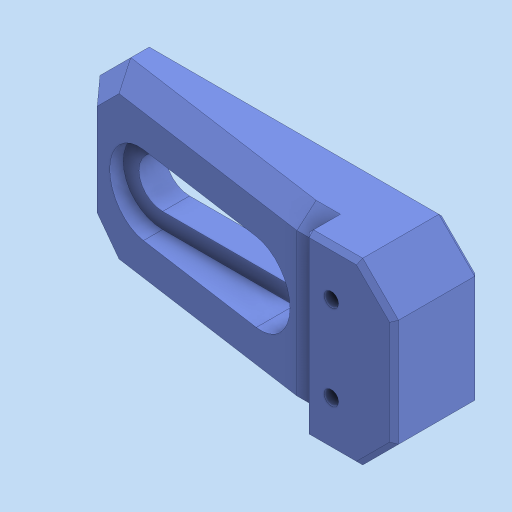
# Autodesk Inventor part: y-Max Endstop Slider for 4040
Saved by Autodesk Inventor 2023.2 (Build 272271000, 271)
## iProperties
Created: 2023-11-28
Part Number: y-Max Endstop Slider for 4040
Material: Generisch
Document SubType Name: Modeling
Designer: Nils Bade
Density: 1 g/cm^3
Appearance: ABS-Blau
Author: Nils Bade
Autodesk Inventor part; units mm, degrees
ref_plane "YZ Plane" through (0, 0, 0) normal (1, 0, 0) x (0, 1, 0)
ref_plane "XZ Plane" through (0, 0, 0) normal (0, 1, 0) x (-1, 0, 0)
ref_plane "XY Plane" through (0, 0, 0) normal (0, 0, 1) x (1, 0, 0)
sketch "S-Base" plane through (0, 0, 0) normal (0, 0, 1) x (1, 0, 0)
  line L0 (-7.35, 0) -> (7.35, 0) construction
  line L1 (-7.35, -2.65) -> (7.35, -2.65)
  line L2 (7.35, 2.65) -> (-7.35, 2.65)
  arc A0 (-7.35, 2.65) -> (-7.35, -2.65) centre (-7.35, 0) ccw
  arc A1 (7.35, -2.65) -> (7.35, 2.65) centre (7.35, 0) ccw
  line L3 (32, 10.3134) -> (32, -10.7721) construction
  line L4 (-24.82, 0) -> (41.47, 0) construction
  circle A2 centre (18, 4.75) radius 0.8
  line L5 (25, 0) -> (25, 10)
  line L6 (25, 10) -> (-15.35, 10)
  line L7 (-15.35, 10) -> (-15.35, 0)
  line L8 (0, 14.5306) -> (0, -14.9892) construction
  line L9 (-7.35, 0) -> (7.35, 0) construction
  line L10 (-7.35, -4.4) -> (7.35, -4.4)
  line L11 (7.35, 4.4) -> (-7.35, 4.4)
  arc A3 (-7.35, 4.4) -> (-7.35, -4.4) centre (-7.35, 0) ccw
  arc A4 (7.35, -4.4) -> (7.35, 4.4) centre (7.35, 0) ccw
  circle A5 centre (18, -4.75) radius 0.8
  line L12 (25, 0) -> (25, -10)
  line L13 (25, -10) -> (-15.35, -10)
  line L14 (-15.35, -10) -> (-15.35, 0)
  line L15 (12.2017, -10) -> (11.9274, 10) construction
  line L16 (15, -10) -> (15, 10)
  point P0 (0, 0)
  point P1 (10, 0)
  point P2 (-10, 0)
  dimension "d0" = 5.3
  dimension "d1" = 20
  dimension "d2" = 22
  dimension "d3" = 1.6
  dimension "d4" = 4.75
  dimension "d5" = 14
  dimension "d6" = 7
  dimension "d7" = 10
  dimension "d8" = 8.8
  dimension "d13" = 6
  dimension "d14" = 8
  dimension "d17" = 3
  constraints: 34 end point, 10 point on circle, 8 tangent, 6 centre point, 6 point on line, 3 perpendicular, 3 symmetric about line, 2 midpoint, 2 parallel, 2 vertical, 1 collinear, 1 horizontal, 1 other
  measures "d0" diameter of A1
  measures "d1" distance of point (10, 0) point (-10, 0)
  measures "d2" distance from line of point (10, 0) L3
  measures "d3" diameter of A2
  measures "d4" distance from line of L4 A2.centre
  measures "d5" distance from line of L3 A2.centre
  measures "d6" distance from line of L5 A2.centre
  measures "d7" distance between parallel lines of L6 L4
  measures "d8" diameter of A4
  measures "d13" distance from line of A2.centre L15
  measures "d14" distance from line of L7 L9.start
  measures "d17" distance from line of A5.centre L16
extrude "Base1" add sketch "S-Base" along normal blind 3 contours A2 | L12 L13 L16 L6 L5 | L16 L13 L14 L7 L6 | A3 L11 A4 L10 | A5
extrude "Base2" add sketch "S-Base" along normal blind 8 contours A2 | L12 L13 L16 L6 L5 | L16 L13 L14 L7 L6 | A5
extrude "Bohrungen" cut sketch "S-Base" against normal blind 3 from surface at 8 contours A2 | A5
extrude "Extrusion4" add sketch "S-Base" along normal blind 1.5 from surface at 8 contours L12 L13 L16 L6 L5
chamfer "Fase-optik1" distance 28 distance2 4 1 edges at (-15.35, 0, 8)
chamfer "Fase-4mm" distance 4 angle 45 4 edges at (-15.35, -10, 2) (-15.35, 10, 2) (25, -10, 4.75) (25, 10, 4.75)
chamfer "Fase-2mm" distance 2 angle 45 7 edges at (0.65, -10, 6.2857) (-13.35, -8, 4.2857) (-15.35, 0, 4) (-13.35, 8, 4.2857) (0.65, 10, 6.2857) (13.825, 10, 8) (13.825, -10, 8)
chamfer "Fase-0,5mm" distance 0.5 angle 45 18 edges at (18, -10, 9.5) (23, -8, 9.5) (15, 0, 9.5) (18, 10, 9.5) (23, 8, 9.5) (25, 0, 9.5) (23, 8, 0) (25, 0, 0) (4.825, 10, 0) (23, -8, 0) (4.825, -10, 0) (-13.35, -8, 0) (-15.35, 0, 0) (-13.35, 8, 0) (15, 10, 7) (15, 10, 8.75) (15, -10, 7) (15, -10, 8.75)
